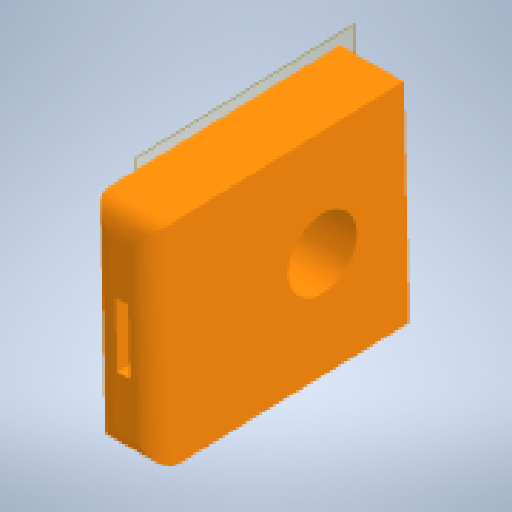
# Autodesk Inventor part: хвост
Saved by Autodesk Inventor 2024.2 (Build 282272000, 272)
## iProperties
Created: 2026-04-03
Part Number: хвост
Material: Типовые
Document SubType Name: Modeling
Designer: katya_notebook
Density: 1 g/cm^3
Appearance: Оранжевый
Author: katya_notebook
Autodesk Inventor part; units mm, degrees
ref_plane "YZ Plane" through (0, 0, 0) normal (1, 0, 0) x (0, 1, 0)
ref_plane "XZ Plane" through (0, 0, 0) normal (0, 1, 0) x (-1, 0, 0)
ref_plane "XY Plane" through (0, 0, 0) normal (0, 0, 1) x (1, 0, 0)
ref_plane "РабПлоскость1" through (-185.8888, -38.5334, 331.0061) normal (0.9999756, 0.0023998, -0.0065586) x (-0.0066118, 0.0228778, -0.9997164)
sketch "Эскиз9" plane through (-185.8888, -38.5334, 331.0061) normal (0.9999756, 0.0023998, -0.0065586) x (-0.0066118, 0.0228778, -0.9997164)
  circle A0 centre (-0.0036, 0) radius 3.25 projected
  line L0 (7.9964, 10) -> (7.9964, -10) projected
  line L1 (7.9964, 10) -> (-0.0036, 10) projected
  arc A1 (-0.0036, 10) -> (-0.0036, -10) centre (-0.0036, 0) ccw projected
  line L2 (-0.0036, -10) -> (7.9964, -10) projected
  line L3 (-0.0036, 10) -> (-16.0036, 10)
  line L4 (-0.0036, -10) -> (-16.0036, -10)
  line L5 (-16.0036, 10) -> (-16.0036, -10)
  point P0 (330.5647, 30.5274)
  point P1 (-10.0036, 0)
  dimension "d24" = 16
  constraints: 6 end point, 2 horizontal, 1 perpendicular
  measures "d24" distance of L1.end L3.end
extrude "Выдавливание4" add sketch "Эскиз9" along normal blind 6
sketch "Эскиз10" plane through (-185.7605, -48.8969, 346.7762) normal (0.0066118, -0.0228778, 0.9997164) x (0.9999756, 0.0023998, -0.0065586)
  line L0 (0, 20) -> (0, 0) projected
  line L1 (0, 0) -> (6, 0) projected
  line L2 (6, 20) -> (6, 0) projected
  line L3 (0, 20) -> (6, 20) projected
  line L4 (0, 20) -> (6, 0)
  line L5 (0, 0) -> (6, 20)
  line L6 (2.4, 6.9) -> (3.6, 6.9)
  line L7 (3.6, 6.9) -> (3.6, 13.1)
  line L8 (3.6, 13.1) -> (2.4, 13.1)
  line L9 (2.4, 13.1) -> (2.4, 6.9)
  line L10 (2.4, 6.9) -> (3.6, 13.1) construction
  line L11 (3.6, 6.9) -> (2.4, 13.1) construction
  point P0 (188.1477, 40.5274)
  point P1 (3, 10)
  dimension "d25" = 1.2
  dimension "d26" = 6.2
  constraints: 16 end point, 3 midpoint, 2 parallel, 1 horizontal, 1 perpendicular
  measures "d25" distance of L7.end L8.end
  measures "d26" distance of L8.end L6.start
extrude "Выдавливание5" cut sketch "Эскиз10" against normal blind 6 contours L9 L8 L7 L5 L4 | L4 L5 L9 | L5 L4 L7 L6 L9 | L7 L4 L5
fillet "Сопряжение1" radius 2 4 edges at (-182.8056, -28.895, 347.2144) (-185.783, -38.8996, 347.0052) (-179.7831, -38.8852, 346.9658) (-182.7606, -48.8897, 346.7565)
